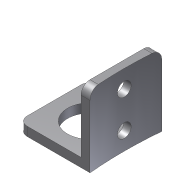
# Autodesk Inventor part: HopperMount
Saved by Autodesk Inventor 2012 (Build 160160000, 160)
## iProperties
Created: 2013-01-23
Part Number: HopperMount
Material: Default
Document SubType Name: Modeling
Designer: JesseK
Density: 1 g/cm^3
Author: JesseK
Autodesk Inventor part; units mm, degrees
ref_plane "YZ Plane" through (0, 0, 0) normal (1, 0, 0) x (0, 1, 0)
ref_plane "XZ Plane" through (0, 0, 0) normal (0, 1, 0) x (-1, 0, 0)
ref_plane "XY Plane" through (0, 0, 0) normal (0, 0, 1) x (1, 0, 0)
sketch "Sketch1" plane through (0, 0, 0) normal (0, 0, 1) x (1, 0, 0)
  line L0 (0, 0) -> (25.4, 0)
  line L1 (25.4, 0) -> (25.4, 25.4)
  line L2 (25.4, 25.4) -> (22.225, 25.4)
  line L3 (22.225, 25.4) -> (22.225, 3.175)
  line L4 (22.225, 3.175) -> (0, 3.175)
  line L5 (0, 3.175) -> (0, 0)
  dimension "d0" = 3.175
  dimension "d1" = 25.4
  constraints: 12 end point, 3 horizontal, 3 vertical, 2 perpendicular
  measures "d0" distance of L4.end L0.start
  measures "d1" distance of L0.start L0.end
extrude "Extrusion1" add sketch "Sketch1" along normal blind 25.4
sketch "Sketch2" plane through (25.4, 0, 0) normal (1, 0, 0) x (0, 0, -1)
  line L0 (0, 0) -> (0, 25.4) projected
  line L1 (0, 25.4) -> (-25.4, 25.4) projected
  circle A0 centre (-12.7, 19.05) radius 2.4384
  circle A1 centre (-12.7, 6.35) radius 2.4384
  line L2 (-12.7, 19.05) -> (-12.7, 6.35) construction
  dimension "d4" = 4.8768
  dimension "d5" = 4.8768
  dimension "d6" = 12.7
  dimension "d7" = 12.7
  dimension "d8" = 6.35
  constraints: 2 centre point, 2 end point, 1 vertical
  measures "d4" diameter of A0
  measures "d5" diameter of A1
  measures "d6" distance between parallel lines of L0 L2
  measures "d7" distance of L2.start L2.end
  measures "d8" distance from line of L1 L2.start
extrude "Extrusion2" cut sketch "Sketch2" against normal through all
sketch "Sketch3" plane through (0, 3.175, 0) normal (0, 1, 0) x (1, 0, 0)
  line L0 (0, -25.4) -> (22.225, -25.4) projected
  line L1 (0, 0) -> (0, -25.4) projected
  circle A0 centre (12.7, -12.7) radius 7.9375
  dimension "d11" = 12.7
  dimension "d12" = 12.7
  dimension "d13" = 15.875
  constraints: 1 centre point
  measures "d11" distance from line of L1 A0.centre
  measures "d12" distance from line of L0 A0.centre
  measures "d13" diameter of A0
extrude "Extrusion3" cut sketch "Sketch3" against normal up to next
fillet "Fillet1" radius 3.175 4 edges at (0, 1.5875, 0) (0, 1.5875, 25.4) (23.8125, 25.4, 25.4) (23.8125, 25.4, 0)
sketch "Sketch4" plane through (25.4, 0, 0) normal (0, -1, 0) x (1, 0, 0)
  line L0 (0, 0) -> (0, 25.4) projected
  arc A0 (0, 25.4) -> (0, 0) centre (139.1215, 12.7) ccw
  line L1 (0, 25.4) -> (0, 0)
  point P0 (-25.4, 0)
  dimension "d17" = 139.7
  constraints: 2 end point, 2 point on circle, 1 centre point, 1 vertical
  measures "d17" radius of A0
extrude "Extrusion4" cut sketch "Sketch4" against normal through all
body "Solid1"
